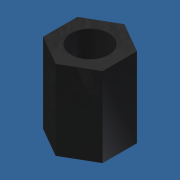
# Autodesk Inventor part: Nutplacer
Saved by Autodesk Inventor 2016 (Build 200138000, 138)
## iProperties
Created: 2015-01-10
Part Number: Nutplacer
Material: ABS-Kunststoff - Schwarz
Document SubType Name: Modeling
Designer: 4ndreas
Density: 1.06 g/cm^3
Appearance: Glatt - weiß(2)
Author: 4ndreas
Autodesk Inventor part; units mm, degrees
ref_plane "YZ Plane" through (0, 0, 0) normal (1, 0, 0) x (0, 1, 0)
ref_plane "XZ Plane" through (0, 0, 0) normal (0, 1, 0) x (-1, 0, 0)
ref_plane "XY Plane" through (0, 0, 0) normal (0, 0, 1) x (1, 0, 0)
sketch "Skizze1" plane through (0, 0, 0) normal (0, 0, 1) x (1, 0, 0)
  line L0 (70.8419, 7.621) -> (77.4419, 3.8105) construction
  line L1 (64.2419, 3.8105) -> (70.8419, 7.621) construction
  line L2 (70.8419, 7.5056) -> (77.3419, 3.7528)
  line L3 (77.3419, 3.7528) -> (77.3419, -3.7528)
  line L4 (77.3419, -3.7528) -> (70.8419, -7.5056)
  line L5 (70.8419, -7.5056) -> (64.3419, -3.7528)
  line L6 (64.3419, -3.7528) -> (64.3419, 3.7528)
  line L7 (64.3419, 3.7528) -> (70.8419, 7.5056)
  circle A0 centre (70.8419, 0) radius 4.1
  point P0 (0, 0)
  dimension "d0" = 13
  dimension "d1" = 8.2
  constraints: 12 end point, 2 coincident, 1 centre point, 1 parallel, 14 other
  measures "d0" distance between parallel lines of L3 L6
  measures "d1" diameter of A0
extrude "Extrusion1" add sketch "Skizze1" against normal blind 8.7
mirror "Spiegeln1" about plane through (70.8419, 0, 0) normal (0, 0, 1) of "Extrusion1"
